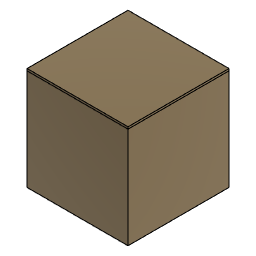
Stone empty v3 (Autodesk Fusion 360 design; units mm, degrees)
Autodesk Fusion 360 part; units mm, degrees
sketch "Skizze1" plane through (0, 0, 0) normal (0, 0, 1) x (1, 0, 0)
  line L0 (0, 0) -> (50, 0)
  line L1 (50, 0) -> (50, 50)
  line L2 (50, 50) -> (0, 50)
  line L3 (0, 50) -> (0, 0)
  line L4 (20, 20) -> (5, 20)
  line L5 (5, 20) -> (5, 5)
  line L6 (5, 5) -> (20, 5)
  line L7 (20, 5) -> (20, 20)
  line L8 (20, 40) -> (35, 40)
  line L9 (35, 40) -> (35, 25)
  line L10 (35, 25) -> (30, 25)
  line L11 (30, 25) -> (30, 30)
  line L12 (30, 30) -> (20, 30)
  line L13 (20, 30) -> (20, 40)
  line L14 (5, 45) -> (15, 45)
  line L15 (15, 45) -> (15, 35)
  line L16 (15, 35) -> (5, 35)
  line L17 (5, 35) -> (5, 45)
  line L18 (30, 15) -> (40, 15)
  line L19 (40, 15) -> (40, 5)
  line L20 (40, 5) -> (30, 5)
  line L21 (30, 5) -> (30, 15)
  line L22 (40, 40) -> (45, 40)
  line L23 (45, 40) -> (45, 30)
  line L24 (45, 30) -> (40, 30)
  line L25 (40, 30) -> (40, 40)
  constraint coincident L0.start L3.end
  constraint horizontal L4
  constraint vertical L5
  constraint horizontal L6
  constraint vertical L7
  constraint horizontal L8
  constraint perpendicular L8 L9
  constraint perpendicular L9 L10
  constraint perpendicular L10 L11
  constraint perpendicular L11 L12
  constraint perpendicular L12 L13
  constraint coincident L8.start L13.end
  constraint horizontal L14
  constraint vertical L15
  constraint horizontal L16
  constraint vertical L17
  constraint horizontal L18
  constraint vertical L19
  constraint horizontal L20
  constraint vertical L21
  constraint horizontal L22
  constraint vertical L23
  constraint horizontal L24
  constraint vertical L25
extrude "Extrusion1" add sketch "Skizze1" along normal blind 25 contours L4 L5 L6 L7 makes body 1 in component "Großer Block"
extrude "Extrusion1'" add sketch "Skizze1" along normal blind 15 separate body contours L18 L19 L20 L21 makes body 2 in component "Medium Block 1"
extrude "Extrusion1''" add sketch "Skizze1" along normal blind 15 separate body contours L14 L15 L16 L17 makes body 3 in component "Medium Block 2#"
extrude "Extrusion1'''" add sketch "Skizze1" along normal blind 10 separate body contours L8 L9 L10 L11 L12 L13 makes body 4 in component "L Block"
extrude "Extrusion1''''" add sketch "Skizze1" along normal blind 5 separate body contours L22 L23 L24 L25 makes body 5 in component "Smal Block 1"
extrude "Extrusion1'''''" add sketch "Skizze1" against normal blind 1 separate body contours L0 L1 L2 L3 | L4 L5 L6 L7 | L8 L9 L10 L11 L12 L13 | L14 L15 L16 L17 | L18 L19 L20 L21 | L22 L23 L24 L25 makes body 6 in component "Boden"
extrude "Extrusion1''''''" add 1 faces at (16.6667, 33.3333, -1) along direction (0, 0, -1) blind 50 separate body on bodies 6 makes body 7 in component "Ground below"
component "Großer Block" placed x (1, 0, 0) y (0, 1, 0) z (0, 0, 1) at (0, 0, 0)
component "Medium Block 1" placed x (1, 0, 0) y (0, 1, 0) z (0, 0, 1) at (0, 0, 0)
component "Medium Block 2#" placed x (1, 0, 0) y (0, 1, 0) z (0, 0, 1) at (0, 0, 0)
component "L Block" placed x (1, 0, 0) y (0, 1, 0) z (0, 0, 1) at (0, 0, 0)
component "Smal Block 1" placed x (1, 0, 0) y (0, 1, 0) z (0, 0, 1) at (0, 0, 0)
component "Boden" placed x (1, 0, 0) y (0, 1, 0) z (0, 0, 1) at (0, 0, 0)
component "Ground below" placed x (1, 0, 0) y (0, 1, 0) z (0, 0, 1) at (0, 0, 0)
